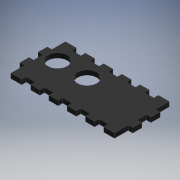
# Autodesk Inventor part: front
Saved by Autodesk Inventor 2019 (Build 230136000, 136)
## iProperties
Created: 2018-06-06
Part Number: front
Material: PBT Plastic Black
Document SubType Name: Modeling
Designer: stra92745
Density: 1.31 g/cm^3
Appearance: Smooth - White
Author: stra92745
Autodesk Inventor part; units mm, degrees
ref_plane "YZ Plane" through (0, 0, 0) normal (1, 0, 0) x (0, 1, 0)
ref_plane "XZ Plane" through (0, 0, 0) normal (0, 1, 0) x (-1, 0, 0)
ref_plane "XY Plane" through (0, 0, 0) normal (0, 0, 1) x (1, 0, 0)
sketch "Sketch1" plane through (0, 0, 0) normal (0, 1, 0) x (-1, 0, 0)
  line L0 (0, 0) -> (-99, 0)
  line L1 (-99, 0) -> (-99, -48)
  line L2 (-99, -48) -> (0, -48)
  line L3 (0, -48) -> (0, 0)
  circle A0 centre (-15, -30) radius 8.5
  circle A1 centre (-41, -30) radius 8.5
  line L4 (-15, -30) -> (-41, -30) construction
  dimension "d0" = 99
  dimension "d1" = 48
  dimension "d2" = 17
  dimension "d3" = 15
  dimension "d4" = 30
  dimension "d5" = 26
  constraints: 10 end point, 2 centre point, 2 horizontal, 2 parallel, 1 equal radius, 1 perpendicular
  measures "d0" distance of L2.end L1.end
  measures "d1" distance of L1.end L0.end
  measures "d2" diameter of A0
  measures "d3" distance from line of L3 L4.start
  measures "d4" distance from line of L0 L4.start
  measures "d5" distance of L4.start L4.end
extrude "Extrusion1" add sketch "Sketch1" along normal blind 4
sketch "Sketch2" plane through (0, 4, 0) normal (0, 1, 0) x (1, 0, 0)
  line L0 (99, 48) -> (0, 48) construction
  line L1 (99, 0) -> (99, 48) construction
  line L2 (0, 0) -> (99, 0) construction
  line L3 (0, 48) -> (0, 0) construction
  line L4 (4, 44) -> (95, 44) construction
  line L5 (95, 44) -> (95, 4) construction
  line L6 (95, 4) -> (4, 4) construction
  line L7 (4, 4) -> (4, 44) construction
  line L8 (4, 36) -> (0, 36)
  line L9 (0, 36) -> (0, 48)
  line L10 (0, 48) -> (4, 48)
  line L11 (4, 48) -> (4, 36)
  line L12 (0, 24) -> (99, 24) construction
  line L13 (49.5, 0) -> (49.5, 48) construction
  line L14 (0, 28) -> (4, 28)
  line L15 (0, 28) -> (0, 24)
  line L16 (4, 28) -> (4, 24)
  line L17 (13.5, 48) -> (13.5, 44)
  line L18 (13.5, 44) -> (21.5, 44)
  line L19 (21.5, 44) -> (21.5, 48)
  line L20 (21.5, 48) -> (13.5, 48)
  line L21 (29.5, 48) -> (29.5, 44)
  line L22 (29.5, 44) -> (37.5, 44)
  line L23 (37.5, 48) -> (37.5, 44)
  line L24 (37.5, 48) -> (29.5, 48)
  line L25 (45.5, 44) -> (45.5, 48)
  line L26 (45.5, 44) -> (49.5, 44)
  line L27 (49.5, 48) -> (45.5, 48)
  line L28 (4, 12) -> (0, 12)
  line L29 (0, 12) -> (0, 0)
  line L30 (0, 0) -> (4, 0)
  line L31 (4, 0) -> (4, 12)
  line L32 (0, 20) -> (4, 20)
  line L33 (0, 20) -> (0, 24)
  line L34 (4, 20) -> (4, 24)
  line L35 (13.5, 0) -> (13.5, 4)
  line L36 (13.5, 4) -> (21.5, 4)
  line L37 (21.5, 4) -> (21.5, 0)
  line L38 (21.5, 0) -> (13.5, 0)
  line L39 (29.5, 0) -> (29.5, 4)
  line L40 (29.5, 4) -> (37.5, 4)
  line L41 (37.5, 0) -> (37.5, 4)
  line L42 (37.5, 0) -> (29.5, 0)
  line L43 (45.5, 4) -> (45.5, 0)
  line L44 (45.5, 4) -> (49.5, 4)
  line L45 (49.5, 0) -> (45.5, 0)
  line L46 (99, 48) -> (99, 0) construction
  line L47 (95, 4) -> (95, 44) construction
  line L48 (95, 36) -> (99, 36)
  line L49 (99, 36) -> (99, 48)
  line L50 (99, 48) -> (95, 48)
  line L51 (95, 48) -> (95, 36)
  line L52 (99, 28) -> (95, 28)
  line L53 (99, 28) -> (99, 24)
  line L54 (95, 28) -> (95, 24)
  line L55 (85.5, 48) -> (85.5, 44)
  line L56 (85.5, 44) -> (77.5, 44)
  line L57 (77.5, 44) -> (77.5, 48)
  line L58 (77.5, 48) -> (85.5, 48)
  line L59 (69.5, 48) -> (69.5, 44)
  line L60 (69.5, 44) -> (61.5, 44)
  line L61 (61.5, 48) -> (61.5, 44)
  line L62 (61.5, 48) -> (69.5, 48)
  line L63 (53.5, 44) -> (53.5, 48)
  line L64 (53.5, 44) -> (49.5, 44)
  line L65 (49.5, 48) -> (53.5, 48)
  line L66 (99, 0) -> (95, 0)
  line L67 (69.5, 0) -> (69.5, 4)
  line L68 (69.5, 4) -> (61.5, 4)
  line L69 (61.5, 0) -> (69.5, 0)
  line L70 (61.5, 0) -> (61.5, 4)
  line L71 (53.5, 4) -> (53.5, 0)
  line L72 (53.5, 4) -> (49.5, 4)
  line L73 (49.5, 0) -> (53.5, 0)
  line L74 (95, 0) -> (95, 12)
  line L75 (95, 12) -> (99, 12)
  line L76 (99, 12) -> (99, 0)
  line L77 (85.5, 0) -> (85.5, 4)
  line L78 (99, 20) -> (95, 20)
  line L79 (77.5, 0) -> (85.5, 0)
  line L80 (77.5, 4) -> (77.5, 0)
  line L81 (85.5, 4) -> (77.5, 4)
  line L82 (95, 20) -> (95, 24)
  line L83 (99, 20) -> (99, 24)
  dimension "d8" = 4
  dimension "d11" = 8
  dimension "d12" = 4
  dimension "d14" = 8
  dimension "d15" = 8
  dimension "d16" = 8
  dimension "d17" = 4
  dimension "d18" = 8
  constraints: 160 end point, 49 symmetric about line, 18 point on line, 8 midpoint, 5 perpendicular, 3 collinear, 2 horizontal, 2 vertical, 1 parallel, 11 other
  measures "d11" distance between parallel lines of L14 L8
  measures "d12" distance of L14.start L15.end
  measures "d14" distance of L17.end L18.end
  measures "d15" distance between parallel lines of L21 L19
  measures "d16" distance of L21.end L22.end
  measures "d17" distance of L25.start L26.end
  measures "d18" distance between parallel lines of L23 L25
extrude "Extrusion2" cut sketch "Sketch2" against normal up to surface (4 mm away)
body "Solid1"
